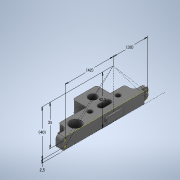
# Autodesk Inventor part: MotorBracket
Saved by Autodesk Inventor 2022 (Build 260153000, 153)
## iProperties
Created: 2021-09-27
Part Number: MotorBracket
Material: 一般
Document SubType Name: Modeling
Designer: shiok
Density: 1 g/cm^3
Appearance: 既定
Author: shiok
Autodesk Inventor part; units mm, degrees
ref_plane "YZ Plane" through (0, 0, 0) normal (1, 0, 0) x (0, 1, 0)
ref_plane "XZ Plane" through (0, 0, 0) normal (0, 1, 0) x (-1, 0, 0)
ref_plane "XY Plane" through (0, 0, 0) normal (0, 0, 1) x (1, 0, 0)
sketch "スケッチ2" plane through (0, 0, 0) normal (0, 1, 0) x (-1, 0, 0)
  circle A0 centre (5.3995, -6) radius 6.15 construction
  circle A1 centre (-4.5, -18.25) radius 9.6 construction
  circle A2 centre (-4.5, 6.25) radius 9.6 construction
  circle A3 centre (-7.3, 21.7491) radius 6.15 construction
  line L0 (12.5, 29) -> (-12.5, 29)
  line L1 (-12.5, -29) -> (12.5, -29)
  line L2 (12.5, -29) -> (12.5, 29)
  circle A4 centre (-4.5, 6.25) radius 11 construction
  circle A5 centre (-4.5, -18.25) radius 11 construction
  line L3 (-4.5, -4.75) -> (-4.5, -7.25) construction
  circle A6 centre (-7.3, 21.7491) radius 5
  line L4 (-12.5, 29) -> (-14.1, 29) construction
  line L5 (-14.1, 29) -> (-14.1, -29) construction
  line L6 (-14.1, -29) -> (-12.5, -29) construction
  circle A7 centre (-4.5, 6.25) radius 2
  circle A8 centre (-4.5, -18.25) radius 2
  circle A9 centre (5.3995, -6) radius 2 construction
  circle A10 centre (-7.3, 21.7491) radius 2
  line L7 (-1.4479, 21.7491) -> (-8.1698, 21.7491)
  circle A11 centre (5.3995, -6) radius 3.5
  circle A12 centre (-4.5, -18.25) radius 3.5 construction
  circle A13 centre (-4.5, 6.25) radius 3.5 construction
  line L8 (-12.5, 29) -> (12.5, -29) construction
  line L9 (12.5, 29) -> (-12.5, -29) construction
  line L10 (-7.3, 26.7491) -> (-7.3, 29) construction
  line L11 (-12.5, -29) -> (-12.5, 29)
  line L12 (-12.5, 21.7491) -> (-12.3, 21.7491) construction
  point P0 (0, 0)
  point P1 (-7.3, 25.2491)
  point P2 (-7.3, 18.2491)
  point P3 (0, 0)
  point P4 (0, 0)
  point P5 (-15.2978, -6)
  dimension "d12" = 22
  dimension "d13" = 22
  dimension "d4" = 12.3
  dimension "d5" = 12.3
  dimension "d6" = 19.2
  dimension "d7" = 19.2
  dimension "d14" = 2.5
  dimension "d15" = 10
  dimension "d16" = 1.6
  dimension "d17" = 4
  dimension "d18" = 4
  dimension "d19" = 4
  dimension "d20" = 4
  dimension "d23" = 7
  dimension "d24" = 7
  dimension "d25" = 7
  dimension "d26" = 7
  dimension "d183" = 58
  dimension "d184" = 23
  dimension "d189" = 9.6
  dimension "d192" = 0.2
  dimension "d208" = 25
  constraints: 26 end point, 12 centre point, 12 coincident, 7 point on line, 5 perpendicular, 4 vertical alignment, 3 horizontal, 3 tangent, 2 midpoint, 2 parallel, 2 point on circle, 1 horizontal alignment, 1 symmetric about line, 5 other
  measures "d4" diameter of A0
  measures "d5" diameter of A3
  measures "d6" diameter of A2
  measures "d7" diameter of A1
  measures "d14" distance of L3.start L3.end
  measures "d15" diameter of A6
  measures "d16" distance of L1.start L5.end
  measures "d17" diameter of A7
  measures "d18" diameter of A8
  measures "d19" diameter of A9
  measures "d20" diameter of A10
  measures "d23" distance of point (-7.3, 18.249) point (-7.3, 25.249)
  measures "d24" diameter of A11
  measures "d25" diameter of A12
  measures "d26" diameter of A13
  measures "d183" distance between parallel lines of L0 L1
  measures "d184" distance from line of L1 point (-15.298, -6)
  measures "d189" distance from line of L5 point (-4.5, -18.25)
  measures "d192" distance of L12.start L12.end
  measures "d208" distance of L1.start L1.end
extrude "押し出し1" add sketch "スケッチ2" along normal blind 10 contours L2 L1 L11 L0
sketch "スケッチ5" plane through (0, 10, 0) normal (0, 1, 0) x (1, 0, 0)
  circle A0 centre (7.3, -21.7491) radius 5
  circle A1 centre (7.3, -21.7491) radius 2
  circle A2 centre (7.3, -21.7491) radius 5 projected
  point P0 (0, 0)
  point P1 (12.0247, -19.5445)
  point P2 (12.0247, -23.6905)
  dimension "d48" = 10
  constraints: 1 centre point, 4 other
extrude "押し出し2" add sketch "スケッチ5" along normal blind 1 from surface at -10
sketch "スケッチ7" plane through (0, 0, 0) normal (0, -1, 0) x (1, 0, 0)
  circle A0 centre (7.3, 21.7491) radius 3.5 construction
  circle A1 centre (7.3, 21.7491) radius 2
  circle A2 centre (7.3, 21.7491) radius 2 projected
  point P0 (0, 0)
  point P1 (7.3, 18.2491)
  point P2 (7.3, 25.2491)
  dimension "d61" = 7
  constraints: 2 centre point, 2 concentric, 2 point on circle, 2 vertical alignment
  measures "d61" diameter of A0
hole "穴1" at (7.3, 0, 18.2491) at (7.3, 0, 25.2491) direction (0, 1, 0) diameter 1.8 end through all countersink diameter 3.6 countersink angle 90 clearance for "Countersunk Flat Head Screw ISO 2009/7046" size "M1.6" standard "ISO"
sketch "スケッチ8" plane through (0, 10, 0) normal (0, 1, 0) x (1, 0, 0)
  line L0 (-12.5, -29) -> (12.5, -29) projected
  line L1 (12.5, -29) -> (7.5, -29)
  line L2 (7.5, -29) -> (7.5, -39)
  line L3 (7.5, -39) -> (12.5, -39)
  line L4 (12.5, -39) -> (12.5, -29)
  line L5 (-11.6501, 0) -> (9.0657, 0)
  line L6 (12.5, 29) -> (7.5, 29)
  line L7 (7.5, 29) -> (7.5, 39)
  line L8 (7.5, 39) -> (12.5, 39)
  line L9 (12.5, 39) -> (12.5, 29)
  point P0 (0, 0)
  point P1 (0.7901, -27.8087)
  dimension "d70" = 5
  dimension "d71" = 10
  constraints: 18 end point, 4 symmetric about line, 3 horizontal, 2 parallel, 1 perpendicular, 1 other
  measures "d70" distance of L3.end L2.end
  measures "d71" distance of L2.end L1.end
extrude "押し出し4" add sketch "スケッチ8" against normal up to surface (10 mm away) contours L0 L4 L3 L2
sketch "スケッチ9" plane through (7.5, 10, 29) normal (-1, 0, 0) x (0, 0, 1)
  line L0 (10, -10) -> (0, -10) projected
  line L1 (10, 0) -> (10, -10) projected
  line L2 (0, 0) -> (10, 0) projected
  line L3 (0, -10) -> (0, 0) projected
  line L4 (10, 0) -> (10, -10) projected
  line L5 (0, -10) -> (10, -10)
  line L6 (10, -10) -> (10, -5)
  line L7 (10, -5) -> (0, -5)
  line L8 (0, -5) -> (0, -10)
  line L9 (10, 0) -> (0, 0)
  line L10 (10, 0) -> (10, -5)
  line L11 (0, -5) -> (0, 0)
  point P0 (7, -7.5)
  point P1 (7, -2.5)
  dimension "d190" = 3
  dimension "d191" = 5
  constraints: 14 end point, 3 symmetric about line, 2 parallel, 1 horizontal, 1 midpoint, 1 perpendicular, 1 vertical alignment
  measures "d190" distance from line of L1 point (7, -7.5)
  measures "d191" distance of point (7, -2.5) point (7, -7.5)
sketch "スケッチ11" plane through (0, 0, 0) normal (0, -1, 0) x (1, 0, 0)
  point P0 (0, 0)
  point P1 (7.5, 29)
  point P2 (7.8247, 0)
hole "穴2" at (7.5, 2.5, 36) at (7.5, 7.5, 36) direction (1, 0, 0) diameter 1.567 end through all thread size "M2x0.4" class "6H" standard "ISO Metric profile"
sketch "スケッチ14" plane through (0, 10, 0) normal (0, 1, 0) x (1, 0, 0)
  line L0 (7.5, 3) -> (7.5, 9)
  line L1 (2.5, 9) -> (2.5, 3)
  line L2 (-17.5, -34) -> (-0.5, -34)
  line L3 (-0.5, -34) -> (-0.5, -4.5)
  line L4 (-0.5, -4.5) -> (-17.5, -4.5)
  line L5 (-17.5, -4.5) -> (-17.5, -34)
  line L6 (-17.5, 16.5) -> (-0.5, 16.5)
  line L7 (-0.5, 16.5) -> (-0.5, 34)
  line L8 (-0.5, 34) -> (-17.5, 34)
  line L9 (-17.5, 34) -> (-17.5, 16.5)
  circle A0 centre (-5.3995, 6) radius 3.5
  circle A1 centre (4.5, 18.25) radius 2
  circle A2 centre (4.5, -6.25) radius 2
  line L10 (12.5, -39.3912) -> (12.5, 29)
  line L11 (-12.5, 29) -> (-12.5, -29)
  line L12 (12.5, 29) -> (-12.5, 29)
  line L13 (-12.5, -29) -> (8.6247, -29)
  arc A3 (2.5, -21.7491) -> (2.5, -21.7491) centre (7.3, -21.7491) ccw
  arc A4 (2.5, 3) -> (7.5, 3) centre (5, 3) ccw
  arc A5 (7.5, 9) -> (2.5, 9) centre (5, 9) ccw
  line L14 (-5.3995, 6) -> (2.5, 6) construction
  circle A6 centre (-5.3995, 6) radius 3.5 projected
  circle A7 centre (4.5, 18.25) radius 2 projected
  circle A8 centre (4.5, -6.25) radius 2 projected
  line L15 (12.5, -39) -> (12.5, 29) projected
  circle A9 centre (7.3, -21.7491) radius 5 projected
  line L16 (12.5, 29) -> (-12.5, 29) projected
  line L17 (-12.5, -29) -> (7.5, -29) projected
  line L18 (-12.5, 29) -> (-12.5, -29) projected
  point P0 (0, 0)
  point P1 (12.8247, -3.7087)
  point P2 (12.5, -39.3912)
  point P3 (12.0247, -19.5445)
  point P4 (12.0247, -23.6905)
  point P5 (-0.5, -29)
  point P6 (-0.5, 29)
  point P7 (-12.5, -4.5)
  point P8 (-12.5, 16.5)
  dimension "d117" = 5
  dimension "d118" = 5
  dimension "d119" = 5
  dimension "d120" = 5
  dimension "d136" = 10.5
  dimension "d137" = 10.5
  dimension "d175" = 6
  dimension "d185" = 5
  dimension "d186" = 4
  dimension "d187" = 4
  dimension "d188" = 7
  dimension "d209" = 13
  constraints: 28 end point, 6 centre point, 6 point on circle, 5 collinear, 5 parallel, 4 horizontal alignment, 4 tangent, 3 concentric, 3 horizontal, 2 coincident, 2 perpendicular, 1 midpoint, 1 vertical alignment, 5 other
  measures "d118" distance between parallel lines of L9 L11
  measures "d119" distance between parallel lines of L8 L12
  measures "d120" distance between parallel lines of L2 L13
  measures "d136" distance from line of L14.start L6
  measures "d137" distance from line of L4 L14.start
  measures "d175" distance of L1.start L1.end
  measures "d185" distance between parallel lines of L1 L0
  measures "d186" diameter of A2
  measures "d187" diameter of A1
  measures "d188" diameter of A0
extrude "押し出し6" cut sketch "スケッチ14" against normal blind 25 contours A4 L1 A5 L0 | L5 L4 L11 L13 L3 L2 | L13 L11 L4 L3 | L9 L8 L7 L12 L11 L6 | L11 L12 L7 L6
sketch "スケッチ15" plane through (0, 0, 0) normal (0, -1, 0) x (1, 0, 0)
  circle A0 centre (4.5, 6.25) radius 2 projected
  circle A1 centre (4.5, 6.25) radius 3
  circle A2 centre (4.5, -18.25) radius 2 projected
  circle A3 centre (4.5, -18.25) radius 3
  point P0 (0, 0)
  dimension "d125" = 6
  dimension "d127" = 6
  constraints: 2 centre point, 2 coincident
  measures "d125" diameter of A1
  measures "d127" diameter of A3
extrude "押し出し7" add sketch "スケッチ15" along normal blind 0.5
fillet "フィレット8" radius 1 2 edges at (1.5, 0, -18.25) (1.5, 0, 6.25)
fillet "フィレット9" radius 2 4 edges at (-0.5, 5, 29) (-12.5, 5, 4.5) (-12.5, 5, -16.5) (-0.5, 5, -29)
fillet "フィレット11" radius 4 1 edges at (7.5, 5, 29)
mirror "ミラー5" about plane through (0, 0, 0) normal (0, 0, 1) of "押し出し4", "穴2", "フィレット11"
fillet "フィレット13" radius 2.5 2 edges at (10, 10, 39) (10, 0, 39)
mirror "ミラー6" about plane through (0, 0, 0) normal (0, 0, 1) of "フィレット13"
sketch "スケッチ18" plane through (7.5, 10, -9) normal (-1, 0, 0) x (0, 0, 1)
  line L0 (6, 0) -> (6, -10) projected
  line L1 (0, 0) -> (6, 0) projected
  point P0 (9, -10)
  point P1 (3, -5)
  point P2 (10.5, 0)
  point P3 (10.5, -10)
  dimension "d164" = 3
  dimension "d165" = 5
  constraints: 1 other
  measures "d165" distance from line of L1 point (3, -5)
hole "穴6" at (7.5, 5, -6) direction (1, 0, 0) diameter 1.567 end through all thread size "M2x0.4" class "6H" standard "ISO Metric profile"
sketch "スケッチ20" plane through (12.5, 2.5, 39) normal (1, 0, 0) x (0, 0, -1)
  circle A0 centre (75, 0) radius 0.7835 construction
  circle A1 centre (75, 5) radius 0.7835 construction
  circle A2 centre (45, 2.5) radius 0.7835 construction
  circle A3 centre (3, 0) radius 0.7835 construction
  circle A4 centre (3, 5) radius 0.7835 construction
  line L0 (75, 0) -> (45, 40) construction
  line L1 (45, 40) -> (3, 0) construction
  line L2 (75, 5) -> (45, 40) construction
  line L3 (3, 5) -> (45, 40) construction
  line L4 (45, -2.5) -> (45, 40) construction
  line L5 (2.5, 7.5) -> (75.5, 7.5) construction
  line L6 (90.9695, -2.5) -> (-0.9695, -2.5) construction
  dimension "d195" = 42.5
  dimension "d196" = 35
  dimension "d197" = 40
  dimension "d198" = 42
  dimension "d199" = 30
  dimension "d200" = 2.5
  constraints: 12 end point, 1 midpoint, 1 point on line, 1 vertical
  measures "d195" distance of L4.start L0.end
  measures "d196" vertical distance of L3.start L0.end
  measures "d197" vertical distance of L1.end L0.end
  measures "d198" horizontal distance of L3.start L0.end
  measures "d199" horizontal distance of L2.start L0.end
  measures "d200" distance from line of L6 L1.end
sketch "スケッチ21" plane through (-0.5, 0, 4.5) normal (-1, 0, 0) x (0, 0, 1)
  line L0 (-21, 0) -> (-31.5, 0) projected
  line L1 (-21, 10) -> (-21, 0) projected
  line L2 (-31.5, 10) -> (-21, 10) projected
  line L3 (22.5, 10) -> (22.5, 0) projected
  line L4 (0, 10) -> (22.5, 10) projected
  line L5 (0, 10) -> (0, 0) projected
  line L6 (22.5, 0) -> (0, 0) projected
  line L7 (-31.5, 0) -> (-31.5, 10) projected
  point P0 (-4.5, 0)
  point P1 (-26.25, 5)
  point P2 (11.25, 5)
  constraints: 2 other
hole "穴7" at (-0.5, 5, 15.75) at (-0.5, 5, -21.75) direction (1, 0, 0) diameter 1.567 depth 6.3 tip angle 118 thread size "M2x0.4" class "6H" standard "ISO Metric profile"
sketch "スケッチ22" plane through (0, 10, 0) normal (0, 1, 0) x (1, 0, 0)
  line L0 (12.5, 39) -> (7.5, 39) projected
  line L1 (12.5, 39) -> (10, 39)
  line L2 (10, 39) -> (10, 33)
  line L3 (10, 33) -> (12.5, 33)
  line L4 (12.5, 33) -> (12.5, 39)
  point P0 (0, 0)
  point P1 (12.5, -39)
  dimension "d212" = 2.5
  dimension "d213" = 6
  constraints: 8 end point, 2 parallel, 1 horizontal, 1 perpendicular
  measures "d212" distance of L3.end L2.end
  measures "d213" distance of L2.end L1.end
extrude "押し出し8" cut sketch "スケッチ22" against normal blind 10
sketch "スケッチ25" plane through (12.5, 2.5, 39) normal (1, 0, 0) x (0, 0, -1)
  line L0 (37.5, 7.5) -> (37.5, -2.5)
  line L1 (52.5, 7.5) -> (52.5, -2.5)
  line L2 (37.5, 5) -> (52.5, 5)
  line L3 (52.5, 5) -> (52.5, 0)
  line L4 (52.5, 0) -> (37.5, 0)
  line L5 (37.5, 0) -> (37.5, 5)
  line L6 (37.5, 5) -> (52.5, 0) construction
  line L7 (52.5, 5) -> (37.5, 0) construction
  circle A0 centre (45, 2.5) radius 0.7835 construction
  line L8 (53.5, 7.5) -> (36.5, 7.5) construction
  line L9 (45, 7.5) -> (45, 5) construction
  line L10 (45, 2.5) -> (45, 0) construction
  line L11 (45, 2.5) -> (45, 5) construction
  line L12 (45, 0) -> (45, -2.5) construction
  line L13 (37.5, -2.5) -> (52.5, -2.5) construction
  line L14 (72, -2.5) -> (2.5, -2.5) projected
  point P0 (45, 2.5)
  dimension "d232" = 15
  constraints: 26 end point, 7 midpoint, 3 collinear, 2 parallel, 2 perpendicular, 2 point on line, 1 coincident, 1 horizontal
  measures "d232" distance between parallel lines of L1 L0
extrude "押し出し11" add sketch "スケッチ25" along normal blind 1.6 contours L2 L1 L4 L0
fillet "フィレット15" radius 2 4 edges at (13.3, 7.5, 1.5) (13.3, 7.5, -13.5) (13.3, 2.5, -13.5) (13.3, 2.5, 1.5)
sketch "スケッチ26" plane through (-12.5, 0, -14.5) normal (-1, 0, 0) x (0, 0, 1)
  line L0 (43.5, 0) -> (14.5, 0)
  line L1 (14.5, 0) -> (14.5, 1.5)
  line L2 (14.5, 1.5) -> (43.5, 1.5)
  line L3 (-14.5, 0) -> (2.5, 0)
  line L4 (2.5, 0) -> (2.5, 1.5)
  line L5 (2.5, 1.5) -> (-14.5, 1.5)
  line L6 (8.5, 0) -> (8.5, 42.5) construction
  line L7 (-14.5, 0) -> (-14.5, 1.5)
  line L8 (43.5, 0) -> (43.5, 1.5)
  line L9 (43.5, 0) -> (43.5, 10) projected
  line L10 (-14.5, 10) -> (-14.5, 0) projected
  line L11 (-2, 0) -> (-12.5, 0) projected
  point P0 (14.5, 0)
  dimension "d238" = 6
  dimension "d243" = 1.5
  constraints: 16 end point, 5 collinear, 3 parallel, 2 horizontal, 2 perpendicular, 1 vertical, 1 other
  measures "d238" distance between parallel lines of L1 L6
  measures "d243" distance between parallel lines of L5 L3
extrude "押し出し12" add sketch "スケッチ26" along normal blind 1.6 and the other way blind 2 from surface at -12
fillet "フィレット18" radius 2 4 edges at (-2.1, 0.75, 29) (-2.1, 0.75, 4.5) (-2.1, 0.75, -16.5) (-2.1, 0.75, -29)
sketch "スケッチ27" plane through (7.5, 0, -33) normal (-1, 0, 0) x (0, 0, 1)
  line L0 (69.5, 10) -> (0, 10) projected
  line L1 (0, 10) -> (-6, 10)
  line L2 (-6, 10) -> (-6, 0)
  line L3 (-6, 0) -> (0, 0)
  line L4 (0, 0) -> (0, 10)
  point P0 (33, 0)
  constraints: 8 end point, 2 parallel, 1 horizontal, 1 perpendicular
extrude "押し出し13" add sketch "スケッチ27" against normal up to surface (2.5 mm away)
fillet "フィレット19" radius 2.5 2 edges at (8.75, 0, -39) (8.75, 10, -39)
sketch "スケッチ28" plane through (10, 0, -33) normal (1, 0, 0) x (0, 0, -1)
  arc A0 (6, 7.5) -> (3.5, 10) centre (3.5, 7.5) ccw projected
  line L0 (0, 10) -> (3.5, 10) projected
  line L1 (0, 10) -> (0, 0) projected
  line L2 (3.5, 0) -> (0, 0) projected
  arc A1 (3.5, 0) -> (6, 2.5) centre (3.5, 2.5) ccw projected
  line L3 (6, 7.5) -> (6, 2.5) projected
  circle A2 centre (3, 7.5) radius 0.7835 construction
  circle A3 centre (3, 2.5) radius 0.7835 construction
  line L4 (3, 7.5) -> (3, 2.5) construction
  point P0 (-33, 0)
  point P1 (3, 5)
  constraints: 2 end point, 1 midpoint, 1 vertical
hole "穴8" at (10, 5, -36) direction (-1, 0, 0) diameter 1.567 depth 6.3 thread size "M2x0.4" class "6H" standard "ISO Metric profile"
